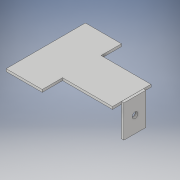
# Autodesk Inventor part: ultrasonic_sensor_ho
Saved by Autodesk Inventor 2017 (Build 210142000, 142)
## iProperties
Created: 2020-01-19
Part Number: ultrasonic_sensor_ho
Material: Generic
Document SubType Name: Modeling
Designer: Admin
Density: 1 g/cm^3
Appearance: Default
Mass: 3.56459 g
Surface Area: 49.119 cm^2
Volume: 3.56459 cm^3
Author: Admin
Autodesk Inventor part; units mm, degrees
ref_plane "YZ Plane" through (0, 0, 0) normal (1, 0, 0) x (0, 1, 0)
ref_plane "XZ Plane" through (0, 0, 0) normal (0, 1, 0) x (-1, 0, 0)
ref_plane "XY Plane" through (0, 0, 0) normal (0, 0, 1) x (1, 0, 0)
sketch "Sketch1" plane through (0, 0, 0) normal (0, 1, 0) x (-1, 0, 0)
  line L0 (-11.5541, -25.4) -> (11.5541, -25.4)
  line L1 (11.5541, -25.4) -> (11.5541, 25.4)
  line L2 (11.5541, 25.4) -> (-11.5541, 25.4)
  line L3 (-11.5541, 25.4) -> (-11.5541, -25.4)
  line L4 (-11.5541, -25.4) -> (11.5541, 25.4) construction
  line L5 (11.5541, -25.4) -> (-11.5541, 25.4) construction
  line L6 (-43.5634, -12.35) -> (-11.5541, -12.35)
  line L7 (-11.5541, -12.35) -> (-11.5541, 12.35)
  line L8 (-11.5541, 12.35) -> (-43.5634, 12.35)
  line L9 (-43.5634, 12.35) -> (-43.5634, -12.35)
  line L10 (-43.5634, -12.35) -> (-11.5541, 12.35) construction
  line L11 (-11.5541, -12.35) -> (-43.5634, 12.35) construction
  point P0 (0, 0)
  point P1 (-27.5588, 0)
  dimension "d0" = 50.8
  constraints: 24 end point, 4 midpoint, 4 parallel, 2 horizontal, 2 perpendicular, 1 point on line
  measures "d0" distance of L0.end L1.end
extrude "Extrusion1" add sketch "Sketch1" along normal mid plane 1.5875
sketch "Sketch2" plane through (43.5634, -0.7937, -12.35) normal (1, 0, 0) x (0, 0, -1)
  line L0 (-4.8431, -19.1223) -> (-18.9376, -19.1223)
  line L1 (-18.9376, -19.1223) -> (-18.9376, 1.5598)
  line L2 (-18.9376, 1.5598) -> (-4.8431, 1.5598)
  line L3 (-4.8431, 1.5598) -> (-4.8431, -19.1223)
  line L4 (-4.8431, -19.1223) -> (-18.9376, 1.5598) construction
  line L5 (-18.9376, -19.1223) -> (-4.8431, 1.5598) construction
  circle A0 centre (-11.8904, -8.7813) radius 1.8384
  point P0 (-12.35, 0.7937)
  constraints: 12 end point, 4 midpoint, 2 parallel, 1 centre point, 1 horizontal, 1 perpendicular
extrude "Extrusion2" add sketch "Sketch2" along normal blind 1.5875
body "Solid1"
